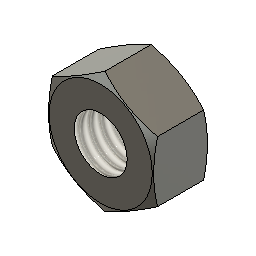
leverextruderalpha (Autodesk Fusion 360 archive; units mm, degrees)
design "Hex Nut Style 1 ANSI B18.2.4.1M - M6 Steel Grade 2H Plain"
description: Hex Nut Style 1 ANSI B18.2.4.1M - M6
part number: HNS1 ANSI B18.2.4.1M - M6 Steel Grade 2H Plain
Autodesk Fusion 360 part; units mm, degrees
sketch "Sketch1" plane through (0, 0, 0) normal (0, 1, 0) x (1, 0, 0)
  line L0 (0, 0) -> (0, -5.2)
  line L1 (-3, 0) -> (-4.9, 0)
  line L2 (-4.9, 0) -> (-5.775, -0.408)
  line L3 (-5.775, -0.408) -> (-5.775, -4.792)
  line L4 (-5.775, -4.792) -> (-4.9, -5.2)
  line L5 (-4.9, -5.2) -> (-3, -5.2)
  line L6 (-3, -5.2) -> (-3, 0)
  dimension "d121" = 6
  dimension "d122" = 25
  dimension "d123" = 25
  dimension "d125" = 9.8
  dimension "d128" = 11.55
  dimension "d153" = 5.2
  constraint vertical L0
  constraint coincident L0 L0.end
  constraint coincident origin L0
  constraint coincident L0.start L1
  constraint coincident L0.start origin
  constraint vertical L1.end L4.end
  constraint coincident L0.end L5
  constraint horizontal L1
  measures "d122" angle of L1 L2
  measures "d123" angle of L4 L5
  measures "d153" distance of L1 L5
revolve "Revolve1" add sketch "Sketch1" angle 360 about axis through (0, 0, 0) along (0, 0, 1)
sketch "Sketch8" plane through (0, 0, 5.2) normal (0, 0, 1) x (1, 0, 0)
  line L0 (-5, -2.8897) -> (-5, 2.8897)
  circle A0 centre (0, 0) radius 3
  circle A1 centre (0, 0) radius 5.775
  dimension "d114" = 5
  constraint coincident L0.end A1
  constraint coincident L0.start A1
  constraint vertical L0
  measures "d114" distance of A0.centre L0
extrude "Extrude5" cut sketch "Sketch8" against normal blind 5.2 contours L0 A1 picked at (-5.125, -0.7039)
pattern_circular "C-Pattern2" count 6 over 360 about axis through (0, 0, 1.75) along (0, 0, 1) of "Extrude5"
thread "Thread3" "ANSI Metric M Profile 6.0 M6x1 M6x1 6H" major diameter 6.147 minor diameter 5.035 pitch 1 angle 60 resizes the face on face at (-2.9963, 0.1495, 3.4667)
equation "adsk_nheig = 5.20 mm"
equation "adsk_maxdia = 11.55 mm"
equation "adsk_nomdia = 6.00 mm"
equation "d89 = -adsk_nheig"
equation "adsk_waflat = 10.00 mm"
equation "d114 = adsk_waflat / 2"
equation "adsk_chamang1 = 25.00 deg"
equation "adsk_chamang2 = 25.00 deg"
equation "d121 = adsk_nomdia"
equation "d122 = adsk_chamang1"
equation "d123 = adsk_chamang2"
equation "d125 = adsk_beardia"
equation "d128 = adsk_maxdia"
equation "d147 = adsk_nheig"
equation "adsk_beardia = adsk_waflat * 0.98"
equation "d153 = adsk_nheig"

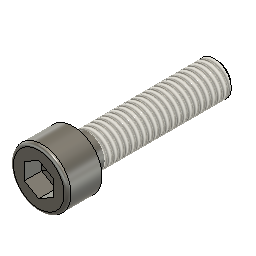
design "Hexagon Socket Head Cap Screw DIN 912 - M6 x 1 x 25 Steel 4.6 Plain"
description: Hexagon Socket Head Cap Screw DIN 912 - M6 x 1 x 25
part number: DIN 912 - M6 x 1 x 25 Steel 4.6 Plain
Autodesk Fusion 360 part; units mm, degrees
sketch "Sketch1" plane through (0, 0, 0) normal (0, 1, 0) x (1, 0, 0)
  line L0 (-3, 0) -> (-3, 25)
  line L1 (-3, 25) -> (0, 25)
  line L2 (0, 25) -> (0, -6)
  line L3 (-3, 0) -> (-5, 0)
  line L4 (-5, 0) -> (-5, -6)
  line L5 (-5, -6) -> (0, -6)
  dimension "d101" = 25
  dimension "d102" = 6
  dimension "d109" = 10
  dimension "d110" = 6
  constraint perpendicular L0 L1
  constraint collinear origin L1.end L2.end
  constraint perpendicular L0 L3
  constraint coincident origin L3
  constraint vertical L2
  constraint coincident L2 L5.end
  constraint perpendicular L2 L5
  measures "d101" distance of origin L1
  measures "d102" distance of L3.end L5
revolve "Revolve1" add sketch "Sketch1" angle 360 about axis through (0, 0, -25) along (0, 0, 1)
ref_plane "WorkPlane1" through (0, 0, 6) normal (0, 0, 1) x (1, 0, 0)
sketch "Sketch6" plane through (0, 0, 6) normal (0, 0, 1) x (1, 0, 0)
  line L0 (0, -2.8868) -> (2.5, -1.4434)
  line L1 (2.5, -1.4434) -> (2.5, 1.4434)
  line L2 (2.5, 1.4434) -> (0, 2.8868)
  line L3 (0, 2.8868) -> (-2.5, 1.4434)
  line L4 (-2.5, 1.4434) -> (-2.5, -1.4434)
  line L5 (-2.5, -1.4434) -> (0, -2.8868)
  dimension "d111" = 5
  constraint vertical L1
  measures "d111" distance of L1 L4
extrude "Extrude1" cut sketch "Sketch6" against normal blind 3
extrude "Extrude2" cut 1 faces at (0, 0.9623, 3) along direction (0, 0, -1) blind 3 draft -85
thread "Thread3" "ISO Metric profile 6.0 M6x1 M6x1 6g" major diameter 5.884 minor diameter 4.7435 pitch 1 angle 60 resizes the face on face at (-2.9851, 0.2987, -16.6667) from (0, 0, -2.5) to (0, 0, -25)
fillet "Fillet4" radius 0.6 1 edges at (-4.6616, 1.8081, 6)
sketch "Sketch7" plane through (0, 0, 0) normal (0, 1, 0) x (1, 0, 0)
  line L0 (-3.06, 25) -> (-3.06, 24.3866)
  line L1 (-3.06, 24.3866) -> (-2.3865, 25)
  line L2 (0, 25) -> (0, -6)
  line L3 (-3.06, 25) -> (0, 25)
  dimension "d104" = 2.3866
  dimension "d105" = 3.06
  dimension "d106" = 0.6135
  constraint coincident L2.start L3.end
  constraint perpendicular L2 L3
  constraint coincident L1.end L3
  constraint perpendicular L0 L3
  measures "d104" distance of L1.end L2
  measures "d105" distance of L0 L2.start
  measures "d106" distance of L0.end L3
revolve "Revolve3" cut sketch "Sketch7" angle 360 about axis through (0, 0, 1.75) along (0, 0, 1)
equation "adsk_nomlen = 25.00 mm"
equation "adsk_headh = 6.00 mm"
equation "adsk_headdia = 10.00 mm"
equation "adsk_nomdia = 6.00 mm"
equation "adsk_philwidth = 5.00 mm"
equation "d31 = -adsk_phildepth"
equation "adsk_phildepth = 3.00 mm"
equation "d71 = adsk_headh"
equation "d76 = -adsk_phildepth"
equation "adsk_thrlen = 22.50 mm"
equation "d86 = adsk_nomdia * 0.1"
equation "adsk_startlen = 0.61345 mm"
equation "adsk_endpointdia = 4.7731 mm"
equation "d101 = adsk_nomlen"
equation "d102 = adsk_headh"
equation "d104 = adsk_endpointdia / 2"
equation "d105 = adsk_nomdia * 0.51"
equation "d106 = adsk_startlen"
equation "d108 = min(adsk_thrlen; adsk_nomlen - 0.001 mm)"
equation "d109 = adsk_headdia"
equation "d110 = adsk_nomdia"
equation "d111 = adsk_philwidth"

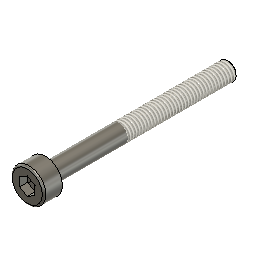
design "Hexagon Socket Head Cap Screw DIN 912 - M3 x 0.5 x 30 Steel 4.6 Plain"
description: Hexagon Socket Head Cap Screw DIN 912 - M3 x 0.5 x 30
part number: DIN 912 - M3 x 0.5 x 30 Steel 4.6 Plain
Autodesk Fusion 360 part; units mm, degrees
sketch "Sketch1" plane through (0, 0, 0) normal (0, 1, 0) x (1, 0, 0)
  line L0 (-1.5, 0) -> (-1.5, 30)
  line L1 (-1.5, 30) -> (0, 30)
  line L2 (0, 30) -> (0, -3)
  line L3 (-1.5, 0) -> (-2.75, 0)
  line L4 (-2.75, 0) -> (-2.75, -3)
  line L5 (-2.75, -3) -> (0, -3)
  dimension "d101" = 30
  dimension "d102" = 3
  dimension "d109" = 5.5
  dimension "d110" = 3
  constraint perpendicular L0 L1
  constraint collinear origin L1.end L2.end
  constraint perpendicular L0 L3
  constraint coincident origin L3
  constraint vertical L2
  constraint coincident L2 L5.end
  constraint perpendicular L2 L5
  measures "d101" distance of origin L1
  measures "d102" distance of L3.end L5
revolve "Revolve1" add sketch "Sketch1" angle 360 about axis through (0, 0, -30) along (0, 0, 1)
ref_plane "WorkPlane1" through (0, 0, 3) normal (0, 0, 1) x (1, 0, 0)
sketch "Sketch6" plane through (0, 0, 3) normal (0, 0, 1) x (1, 0, 0)
  line L0 (0, -1.4434) -> (1.25, -0.7217)
  line L1 (1.25, -0.7217) -> (1.25, 0.7217)
  line L2 (1.25, 0.7217) -> (0, 1.4434)
  line L3 (0, 1.4434) -> (-1.25, 0.7217)
  line L4 (-1.25, 0.7217) -> (-1.25, -0.7217)
  line L5 (-1.25, -0.7217) -> (0, -1.4434)
  dimension "d111" = 2.5
  constraint vertical L1
  measures "d111" distance of L1 L4
extrude "Extrude1" cut sketch "Sketch6" against normal blind 1.3
extrude "Extrude2" cut 1 faces at (0.4167, -0.2406, 1.7) along direction (0, 0, -1) blind 1.3 draft -85
thread "Thread3" "ISO Metric profile 3.0 M3x0.5 M3x0.5 6g" major diameter 2.927 minor diameter 2.3555 pitch 0.5 angle 60 resizes the face on face at (-1.4925, 0.1494, -20) from (0, 0, -12) to (0, 0, -30)
fillet "Fillet4" radius 0.3 1 edges at (-2.5639, 0.9944, 3)
sketch "Sketch7" plane through (0, 0, 0) normal (0, 1, 0) x (1, 0, 0)
  line L0 (-1.53, 30) -> (-1.53, 29.6933)
  line L1 (-1.53, 29.6933) -> (-1.1933, 30)
  line L2 (0, 30) -> (0, -3)
  line L3 (-1.53, 30) -> (0, 30)
  dimension "d104" = 1.1933
  dimension "d105" = 1.53
  dimension "d106" = 0.3067
  constraint coincident L2.start L3.end
  constraint perpendicular L2 L3
  constraint coincident L1.end L3
  constraint perpendicular L0 L3
  measures "d104" distance of L1.end L2
  measures "d105" distance of L0 L2.start
  measures "d106" distance of L0.end L3
revolve "Revolve3" cut sketch "Sketch7" angle 360 about axis through (0, 0, 1.75) along (0, 0, 1)
equation "adsk_nomlen = 30.00 mm"
equation "adsk_headh = 3.00 mm"
equation "adsk_headdia = 5.50 mm"
equation "adsk_nomdia = 3.00 mm"
equation "adsk_philwidth = 2.50 mm"
equation "d31 = -adsk_phildepth"
equation "adsk_phildepth = 1.30 mm"
equation "d71 = adsk_headh"
equation "d76 = -adsk_phildepth"
equation "adsk_thrlen = 18.00 mm"
equation "d86 = adsk_nomdia * 0.1"
equation "adsk_startlen = 0.306725 mm"
equation "adsk_endpointdia = 2.38655 mm"
equation "d101 = adsk_nomlen"
equation "d102 = adsk_headh"
equation "d104 = adsk_endpointdia / 2"
equation "d105 = adsk_nomdia * 0.51"
equation "d106 = adsk_startlen"
equation "d108 = min(adsk_thrlen; adsk_nomlen - 0.001 mm)"
equation "d109 = adsk_headdia"
equation "d110 = adsk_nomdia"
equation "d111 = adsk_philwidth"

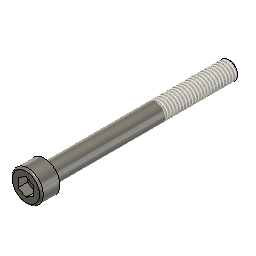
design "Hexagon Socket Head Cap Screw DIN 912 - M6 x 1 x 60 Steel 4.6 Plain"
description: Hexagon Socket Head Cap Screw DIN 912 - M6 x 1 x 60
part number: DIN 912 - M6 x 1 x 60 Steel 4.6 Plain
Autodesk Fusion 360 part; units mm, degrees
sketch "Sketch1" plane through (0, 0, 0) normal (0, 1, 0) x (1, 0, 0)
  line L0 (-3, 0) -> (-3, 60)
  line L1 (-3, 60) -> (0, 60)
  line L2 (0, 60) -> (0, -6)
  line L3 (-3, 0) -> (-5, 0)
  line L4 (-5, 0) -> (-5, -6)
  line L5 (-5, -6) -> (0, -6)
  dimension "d101" = 60
  dimension "d102" = 6
  dimension "d109" = 10
  dimension "d110" = 6
  constraint perpendicular L0 L1
  constraint collinear origin L1.end L2.end
  constraint perpendicular L0 L3
  constraint coincident origin L3
  constraint vertical L2
  constraint coincident L2 L5.end
  constraint perpendicular L2 L5
  measures "d101" distance of origin L1
  measures "d102" distance of L3.end L5
revolve "Revolve1" add sketch "Sketch1" angle 360 about axis through (0, 0, -60) along (0, 0, 1)
ref_plane "WorkPlane1" through (0, 0, 6) normal (0, 0, 1) x (1, 0, 0)
sketch "Sketch6" plane through (0, 0, 6) normal (0, 0, 1) x (1, 0, 0)
  line L0 (0, -2.8868) -> (2.5, -1.4434)
  line L1 (2.5, -1.4434) -> (2.5, 1.4434)
  line L2 (2.5, 1.4434) -> (0, 2.8868)
  line L3 (0, 2.8868) -> (-2.5, 1.4434)
  line L4 (-2.5, 1.4434) -> (-2.5, -1.4434)
  line L5 (-2.5, -1.4434) -> (0, -2.8868)
  dimension "d111" = 5
  constraint vertical L1
  measures "d111" distance of L1 L4
extrude "Extrude1" cut sketch "Sketch6" against normal blind 3
extrude "Extrude2" cut 1 faces at (0.8333, -0.4811, 3) along direction (0, 0, -1) blind 3 draft -85
thread "Thread3" "ISO Metric profile 6.0 M6x1 M6x1 6g" major diameter 5.884 minor diameter 4.7435 pitch 1 angle 60 resizes the face on face at (-2.9851, 0.2987, -40) from (0, 0, -36) to (0, 0, -60)
fillet "Fillet4" radius 0.6 1 edges at (-4.6616, 1.8081, 6)
sketch "Sketch7" plane through (0, 0, 0) normal (0, 1, 0) x (1, 0, 0)
  line L0 (-3.06, 60) -> (-3.06, 59.3866)
  line L1 (-3.06, 59.3866) -> (-2.3865, 60)
  line L2 (0, 60) -> (0, -6)
  line L3 (-3.06, 60) -> (0, 60)
  dimension "d104" = 2.3866
  dimension "d105" = 3.06
  dimension "d106" = 0.6135
  constraint coincident L2.start L3.end
  constraint perpendicular L2 L3
  constraint coincident L1.end L3
  constraint perpendicular L0 L3
  measures "d104" distance of L1.end L2
  measures "d105" distance of L0 L2.start
  measures "d106" distance of L0.end L3
revolve "Revolve3" cut sketch "Sketch7" angle 360 about axis through (0, 0, 1.75) along (0, 0, 1)
equation "adsk_nomlen = 60.00 mm"
equation "adsk_headh = 6.00 mm"
equation "adsk_headdia = 10.00 mm"
equation "adsk_nomdia = 6.00 mm"
equation "adsk_philwidth = 5.00 mm"
equation "d31 = -adsk_phildepth"
equation "adsk_phildepth = 3.00 mm"
equation "d71 = adsk_headh"
equation "d76 = -adsk_phildepth"
equation "adsk_thrlen = 24.00 mm"
equation "d86 = adsk_nomdia * 0.1"
equation "adsk_startlen = 0.61345 mm"
equation "adsk_endpointdia = 4.7731 mm"
equation "d101 = adsk_nomlen"
equation "d102 = adsk_headh"
equation "d104 = adsk_endpointdia / 2"
equation "d105 = adsk_nomdia * 0.51"
equation "d106 = adsk_startlen"
equation "d108 = min(adsk_thrlen; adsk_nomlen - 0.001 mm)"
equation "d109 = adsk_headdia"
equation "d110 = adsk_nomdia"
equation "d111 = adsk_philwidth"
